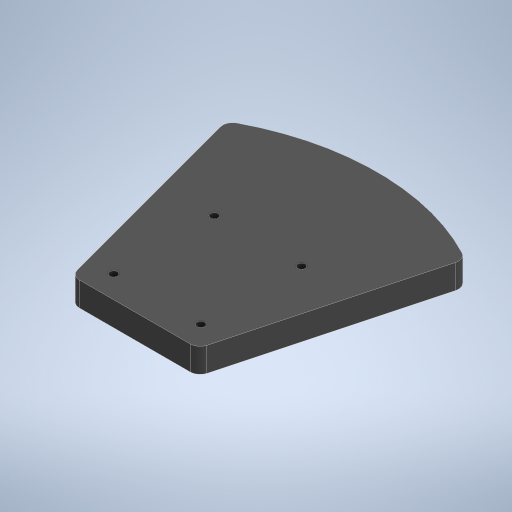
# Autodesk Inventor part: toe_sole_back
Saved by Autodesk Inventor 2024.1 (Build 281209000, 209)
## iProperties
Created: 2024-02-12
Part Number: toe_sole_back
Material: 一般
Document SubType Name: Modeling
Designer: hibik
Density: 1 g/cm^3
Appearance: 既定
Author: hibik
Autodesk Inventor part; units mm, degrees
ref_plane "YZ Plane" through (0, 0, 0) normal (1, 0, 0) x (0, 1, 0)
ref_plane "XZ Plane" through (0, 0, 0) normal (0, 1, 0) x (-1, 0, 0)
ref_plane "XY Plane" through (0, 0, 0) normal (0, 0, 1) x (1, 0, 0)
sketch "スケッチ1" plane through (0, 0, 0) normal (0, 1, 0) x (-1, 0, 0)
  line L0 (26, 0) -> (0, 0)
  line L1 (0, 0) -> (0, -30)
  line L2 (0, -30) -> (26, -30)
  line L3 (26, -30) -> (26, 0)
  line L4 (26, 0) -> (37.6554, -43.4984)
  line L5 (0, 0) -> (-11.6554, -43.4984)
  arc A0 (-11.6554, -43.4984) -> (37.6554, -43.4984) centre (13, 0) ccw
  line L6 (0, 0) -> (26, -30)
  line L7 (0, -30) -> (26, 0)
  line L8 (4, -4.6154) -> (22, -4.6154)
  line L9 (22, -4.6154) -> (22, -25.3846)
  line L10 (22, -25.3846) -> (4, -25.3846)
  line L11 (4, -25.3846) -> (4, -4.6154)
  circle A1 centre (4, -4.6154) radius 0.8
  circle A2 centre (4, -25.3846) radius 0.8
  circle A3 centre (22, -4.6154) radius 0.8
  circle A4 centre (22, -25.3846) radius 0.8
  dimension "d0" = 26
  dimension "d3" = 30
  dimension "d4" = 15
  dimension "d5" = 15
  dimension "d6" = 50
  dimension "d17" = 4
  dimension "d18" = 1.6
  dimension "d19" = 1.6
  dimension "d20" = 1.6
  dimension "d21" = 1.6
  constraints: 24 end point, 6 coincident, 5 centre point, 4 parallel, 3 point on line, 2 horizontal, 2 perpendicular, 2 point on circle, 1 midpoint
  measures "d0" distance of L0.start L0.end
  measures "d3" distance of L2.end L0.start
  measures "d4" angle of L3 L4
  measures "d5" angle of L1 L5
  measures "d6" radius of A0
  measures "d17" distance between parallel lines of L1 L11
  measures "d18" diameter of A1
  measures "d19" diameter of A2
  measures "d20" diameter of A3
  measures "d21" diameter of A4
extrude "押し出し1" add sketch "スケッチ1" along normal blind 4 contours L7 A3 L8 A1 L6 L0 | L4 A0 L5 L1 L2 L3 | L3 L6 A4 L9 A3 L7 | L6 A1 L11 A2 L7 L1 | L2 L7 A2 L10 A4 L6 | A3 L7 L6 A1 L8 | A1 L6 L7 A2 L11 | L10 A2 L7 L6 A4 | A3 L9 A4 L6 L7
sketch "スケッチ2" plane through (0, 0, 0) normal (0, -1, 0) x (1, 0, 0)
  arc A0 (-35.3164, -42.4968) -> (9.3164, -42.4968) centre (-13, 0) ccw
  arc A1 (-37.6554, -43.4984) -> (11.6554, -43.4984) centre (-13, 0) ccw projected
  line L0 (9.3164, -42.4968) -> (6.6453, -32.5279)
  line L1 (-35.3164, -42.4968) -> (-32.6453, -32.5279)
  arc A2 (-32.6453, -32.5279) -> (6.6453, -32.5279) centre (-13, 0) ccw
  line L2 (0, 0) -> (11.6554, -43.4984) projected
  line L3 (-37.6554, -43.4984) -> (-26, 0) projected
  line L4 (-26, 0) -> (0, 0) projected
  circle A3 centre (-4, -4.6154) radius 0.8 projected
  circle A4 centre (-22, -4.6154) radius 0.8 projected
  circle A5 centre (-22, -25.3846) radius 0.8 projected
  circle A6 centre (-4, -25.3846) radius 0.8 projected
  dimension "d9" = 2
  dimension "d10" = 2
  dimension "d11" = 2
  dimension "d12" = 10
  constraints: 4 end point, 4 point on circle, 2 centre point, 2 concentric, 2 parallel
  measures "d9" distance between parallel lines of L2 L0
  measures "d10" distance between parallel lines of L3 L1
  measures "d11" radial gap between concentric circles of A1 A0
  measures "d12" radial gap between concentric circles of A2 A0
extrude "押し出し3" add sketch "スケッチ2" along normal blind 1
fillet "フィレット1" radius 0.5 4 edges at (-13, -1, -38) (7.9808, -1, -37.5123) (-13, -1, -48) (-33.9808, -1, -37.5123)
fillet "フィレット2" radius 2 4 edges at (-37.6554, 1.5, -43.4984) (11.6554, 1.5, -43.4984) (0, 1.5, 0) (-26, 1.5, 0)
sketch "スケッチ3" plane through (0, -1, 0) normal (0, -1, 0) x (1, 0, 0)
  circle A0 centre (-4, -4.6154) radius 0.8 projected
  circle A1 centre (-22, -4.6154) radius 0.8 projected
  circle A2 centre (-22, -25.3846) radius 0.8 projected
  circle A3 centre (-4, -25.3846) radius 0.8 projected
  circle A4 centre (-4, -4.6154) radius 2
  circle A5 centre (-22, -4.6154) radius 2
  circle A6 centre (-22, -25.3846) radius 2
  circle A7 centre (-4, -25.3846) radius 2
  point P0 (0, 0)
  point P1 (-22.7249, -25.7231)
  point P2 (-21.6502, -26.1041)
  point P3 (-4.3498, -26.1041)
  point P4 (-3.2751, -25.7231)
  dimension "d22" = 4
  dimension "d23" = 4
  dimension "d24" = 4
  dimension "d25" = 4
  constraints: 4 centre point, 4 coincident
  measures "d22" diameter of A4
  measures "d23" diameter of A5
  measures "d24" diameter of A6
  measures "d25" diameter of A7
extrude "押し出し4" cut sketch "スケッチ3" against normal blind 2 contours A0 | A1 | A2 | A3 | A4 | A5 | A6 | A7
equation "\"d5\" = d4"
